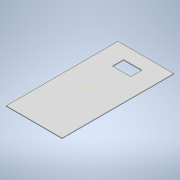
# Autodesk Inventor part: front
Saved by Autodesk Inventor 2021 (Build 250183000, 183)
## iProperties
Created: 2021-03-25
Part Number: front
Material: Generic
Document SubType Name: Modeling
Designer: noori
Density: 1 g/cm^3
Appearance: Default
Author: noori
Autodesk Inventor part; units mm, degrees
ref_plane "YZ Plane" through (0, 0, 0) normal (1, 0, 0) x (0, 1, 0)
ref_plane "XZ Plane" through (0, 0, 0) normal (0, 1, 0) x (-1, 0, 0)
ref_plane "XY Plane" through (0, 0, 0) normal (0, 0, 1) x (1, 0, 0)
sketch "Sketch1" plane through (0, 0, 0) normal (0, 1, 0) x (-1, 0, 0)
  line L0 (200, 400) -> (-200, 400)
  line L1 (-200, 400) -> (-200, -400)
  line L2 (-200, -400) -> (200, -400)
  line L3 (200, -400) -> (200, 400)
  line L4 (65.5, -226.6667) -> (-65.5, -226.6667)
  line L5 (-65.5, -226.6667) -> (-65.5, -306.6667)
  line L6 (-65.5, -306.6667) -> (65.5, -306.6667)
  line L7 (65.5, -306.6667) -> (65.5, -226.6667)
  point P0 (0, 0)
  dimension "d0" = 800
  dimension "d1" = 400
  dimension "d3" = 200
  dimension "d4" = 400
  dimension "d5" = 80
  dimension "d6" = 131
  dimension "d7" = 134.5
  dimension "d8" = 93.3333
  constraints: 16 end point, 4 parallel, 2 horizontal, 2 perpendicular
  measures "d0" distance of L2.end L0.start
  measures "d1" distance of L1.end L2.end
  measures "d3" distance from line of L3 point (0, 0)
  measures "d4" distance from line of L0 point (0, 0)
  measures "d5" distance of L6.end L4.start
  measures "d6" distance of L5.end L6.end
  measures "d7" distance between parallel lines of L3 L7
  measures "d8" distance between parallel lines of L2 L6
sketch "Sketch2" plane through (0, 0, 0) normal (0, 1, 0) x (-1, 0, 0)
  point P0 (0, 0)
sketch "Sketch3" plane through (0, 0, 0) normal (1, 0, 0) x (0, 1, 0)
  point P0 (0, 0)
sketch "Sketch4" plane through (0, 0, 0) normal (0, 1, 0) x (-1, 0, 0)
  point P0 (0, 0)
  point P1 (0, 0)
  constraints: 1 coincident
sketch "Sketch5" plane through (0, 0, 0) normal (0, 1, 0) x (-1, 0, 0)
  point P0 (0, 0)
extrude "Extrusion1" add sketch "Sketch1" along normal mid plane 4
equation "\"d7\" = 0.5 * d1 - 0.5 * d6"
equation "\"d8\" = 0.166667 * d0 - 0.5 * d5"
body "Solid1"
